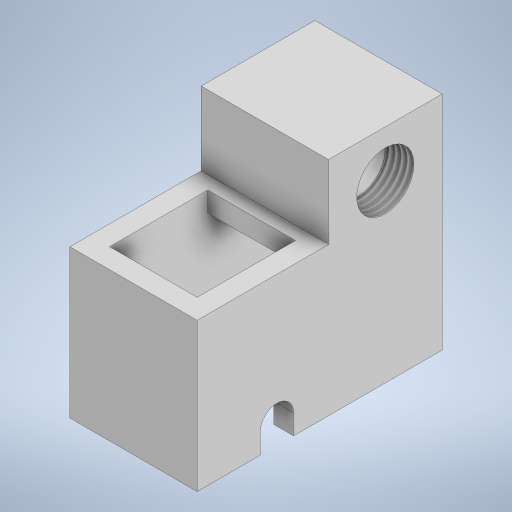
# Autodesk Inventor part: ADAPTER_AOM-brimrose-watercooled-cover-2
Saved by Autodesk Inventor 2024.2 (Build 282272000, 272)
## iProperties
Created: 2024-02-12
Part Number: ADAPTER_AOM-brimrose-watercooled-cover-2
Material: Generic
Document SubType Name: Modeling
Designer: fabig
Density: 1 g/cm^3
Appearance: Default
Author: fabig
Autodesk Inventor part; units mm, degrees
ref_plane "YZ Plane" through (0, 0, 0) normal (1, 0, 0) x (0, 1, 0)
ref_plane "XZ Plane" through (0, 0, 0) normal (0, 1, 0) x (-1, 0, 0)
ref_plane "XY Plane" through (0, 0, 0) normal (0, 0, 1) x (1, 0, 0)
sketch "Sketch1" plane through (0, 0, 0) normal (0, 1, 0) x (-1, 0, 0)
  point P0 (0, 0)
sketch "Sketch2" plane through (0, 0, 0) normal (0, 1, 0) x (-1, 0, 0)
  line L0 (-6.55, 15.35) -> (6.55, 15.35)
  line L1 (6.55, 15.35) -> (6.55, -15.35)
  line L2 (6.55, -15.35) -> (-6.55, -15.35)
  line L3 (-6.55, -15.35) -> (-6.55, 15.35)
  line L4 (-6.55, 15.35) -> (6.55, -15.35) construction
  line L5 (6.55, 15.35) -> (-6.55, -15.35) construction
  line L6 (-9.525, 18.325) -> (9.525, 18.325)
  line L7 (9.525, 18.325) -> (9.525, -18.325)
  line L8 (9.525, -18.325) -> (-9.525, -18.325)
  line L9 (-9.525, -18.325) -> (-9.525, 18.325)
  line L10 (-9.525, 18.325) -> (9.525, -18.325) construction
  line L11 (9.525, 18.325) -> (-9.525, -18.325) construction
  point P0 (0, 0)
  dimension "d0" = 13.1
  dimension "d1" = 30.7
  dimension "d2" = 19.05
  dimension "d3" = 36.65
  constraints: 24 end point, 4 midpoint, 4 parallel, 2 horizontal, 2 perpendicular
  measures "d0" distance of L1.end L2.end
  measures "d1" distance of L0.end L1.end
  measures "d2" distance of L7.end L8.end
  measures "d3" distance of L6.end L7.end
extrude "Extrusion1" add sketch "Sketch2" along normal blind 19.2
sketch "Sketch3" plane through (0, 19.2, 0) normal (0, 1, 0) x (1, 0, 0)
  line L0 (-9.525, -18.325) -> (9.525, -18.325)
  line L1 (9.525, -18.325) -> (9.525, 18.325)
  line L2 (9.525, 18.325) -> (-9.525, 18.325)
  line L3 (-9.525, 18.325) -> (-9.525, -18.325)
  point P0 (0, 0)
  constraints: 8 end point, 2 parallel, 1 horizontal, 1 perpendicular
extrude "Extrusion2" add sketch "Sketch3" along normal blind 3
sketch "Sketch4" plane through (0, 22.2, 0) normal (0, 1, 0) x (1, 0, 0)
  line L0 (-6.55, -15.35) -> (-6.55, 15.35) construction
  line L1 (6.55, -15.35) -> (-6.55, -15.35) construction
  line L2 (-6.55, -15.35) -> (-6.55, 15.35) construction
  line L3 (-6.55, 15.35) -> (6.55, 15.35) construction
  line L4 (6.55, 15.35) -> (6.55, -15.35) construction
  line L5 (6.55, -15.35) -> (-6.55, 15.35) construction
  line L6 (-6.55, -15.35) -> (6.55, 15.35) construction
  line L7 (6.55, 15.35) -> (6.55, -15.35) projected
  line L8 (-6.55, -15.35) -> (6.55, -15.35)
  line L9 (6.55, -15.35) -> (6.55, -0.65)
  line L10 (6.55, -0.65) -> (-6.55, -0.65)
  line L11 (-6.55, -0.65) -> (-6.55, -15.35)
  point P0 (0, 0)
  point P1 (6.55, -15.35)
  dimension "d8" = 14.7
  constraints: 20 end point, 4 parallel, 2 horizontal, 2 midpoint, 2 perpendicular, 1 point on line
  measures "d8" distance of L9.end L8.end
extrude "Extrusion3" cut sketch "Sketch4" against normal blind 5
sketch "Sketch6" plane through (9.525, 0, 18.325) normal (1, 0, 0) x (0, 0, -1)
  line L0 (0, 0) -> (36.65, 0) construction
  line L1 (0, 0) -> (11.925, 0) construction
  line L2 (11.925, 0) -> (11.925, 3) construction
  line L3 (11.925, 3) -> (0, 3) construction
  line L4 (0, 3) -> (0, 0) construction
  circle A0 centre (11.925, 3) radius 2.5
  line L5 (9.425, 3) -> (9.425, -0.2828)
  line L6 (14.425, 3) -> (14.425, 0)
  line L7 (9.425, 0) -> (14.425, 0)
  point P0 (18.325, 0)
  dimension "d16" = 11.925
  dimension "d17" = 3
  dimension "d18" = 5
  constraints: 14 end point, 4 point on line, 3 perpendicular, 2 parallel, 2 point on circle, 2 tangent, 1 centre point, 1 coincident, 1 collinear, 1 horizontal
  measures "d16" distance of L3.end L2.end
  measures "d17" distance of L2.end L1.end
  measures "d18" diameter of A0
extrude "Extrusion5" cut sketch "Sketch6" against normal through all
sketch "Sketch7" plane through (0, 22.2, 0) normal (0, 1, 0) x (1, 0, 0)
  line L0 (9.525, 18.325) -> (-9.525, 18.325) projected
  line L1 (-9.525, 18.325) -> (-9.525, -18.325) projected
  line L2 (9.525, 18.325) -> (-9.525, 18.325)
  line L3 (-9.525, 18.325) -> (-9.525, 1.325)
  line L4 (-9.525, 1.325) -> (9.525, 1.325)
  line L5 (9.525, 1.325) -> (9.525, 18.325)
  point P0 (0, 0)
  dimension "d21" = 17
  constraints: 8 end point, 2 parallel, 1 horizontal, 1 perpendicular, 1 point on line
  measures "d21" distance of L3.end L2.end
extrude "Extrusion6" add sketch "Sketch7" along normal blind 11
sketch "Sketch8" plane through (9.525, 0, 18.325) normal (1, 0, 0) x (0, 0, -1)
  line L0 (19.65, 33.2) -> (36.65, 33.2) construction
  line L1 (28.15, 33.2) -> (28.15, 26.2) construction
  circle A0 centre (28.15, 26.2) radius 4
  point P0 (18.325, 0)
  dimension "d24" = 7
  dimension "d25" = 8
  constraints: 2 end point, 1 centre point, 1 coincident, 1 midpoint, 1 vertical
  measures "d24" distance of L1.start L1.end
  measures "d25" diameter of A0
extrude "Extrusion7" cut sketch "Sketch8" against normal through all
sketch "Sketch9" plane through (9.525, 0, 18.325) normal (1, 0, 0) x (0, 0, -1)
  circle A0 centre (28.15, 26.2) radius 4 construction
  circle A1 centre (28.15, 26.2) radius 4 construction
  point P0 (18.325, 0)
  constraints: 1 centre point, 1 coincident
hole "Hole1" at (9.525, 26.2, -9.825) direction (-1, 0, 0) diameter 8.566 depth 4 thread size "G9.728x0.907" designation "G 1/8" standard "ISO Pipe Threads"
sketch "Sketch10" plane through (-9.525, 0, 18.325) normal (-1, 0, 0) x (0, 0, 1)
  circle A0 centre (-28.15, 26.2) radius 4 construction
  circle A1 centre (-28.15, 26.2) radius 4 construction
  point P0 (-18.325, 0)
  constraints: 1 centre point, 1 coincident
hole "Hole2" at (-9.525, 26.2, -9.825) direction (1, 0, 0) diameter 8.566 depth 4 thread size "G9.728x0.907" designation "G 1/8" standard "ISO Pipe Threads"
body "Solid1"
